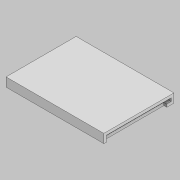
# Autodesk Inventor part: HardDriveCase
Saved by Autodesk Inventor 2021 (Build 250183000, 183)
## iProperties
Created: 2021-03-03
Part Number: HardDriveCase
Material: Generic
Document SubType Name: Modeling
Designer: Merkileg
Density: 1 g/cm^3
Appearance: Default
Author: Merkileg
Autodesk Inventor part; units mm, degrees
ref_plane "YZ Plane" through (0, 0, 0) normal (1, 0, 0) x (0, 1, 0)
ref_plane "XZ Plane" through (0, 0, 0) normal (0, 1, 0) x (-1, 0, 0)
ref_plane "XY Plane" through (0, 0, 0) normal (0, 0, 1) x (1, 0, 0)
sketch "Sketch1" plane through (0, 0, 0) normal (1, 0, 0) x (0, 1, 0)
  line L0 (0, 0) -> (9.779, 0)
  line L1 (9.779, 0) -> (9.779, -77.47)
  line L2 (9.779, -77.47) -> (0, -77.47)
  line L3 (0, -77.47) -> (0, 0)
  line L4 (3.175, -3.175) -> (6.604, -3.175)
  line L5 (6.604, -3.175) -> (6.604, -74.295)
  line L6 (6.604, -74.295) -> (3.175, -74.295)
  line L7 (3.175, -74.295) -> (3.175, -3.175)
  dimension "d0" = 3.175
  dimension "d1" = 3.175
  dimension "d2" = 3.175
  dimension "d3" = 3.175
  dimension "d4" = 3.429
  dimension "d5" = 71.12
  constraints: 16 end point, 4 parallel, 2 horizontal, 2 perpendicular
  measures "d0" distance between parallel lines of L1 L5
  measures "d1" distance between parallel lines of L2 L6
  measures "d2" distance between parallel lines of L0 L4
  measures "d3" distance between parallel lines of L7 L3
  measures "d4" distance between parallel lines of L7 L5
  measures "d5" distance between parallel lines of L6 L4
extrude "Extrusion1" add sketch "Sketch1" along normal blind 104.902
sketch "Sketch2" plane through (0, 0, 0) normal (-1, 0, 0) x (0, 0, 1)
  line L0 (-77.47, 0) -> (-77.47, 9.779) projected
  line L1 (0, 9.779) -> (0, 0) projected
  line L2 (-77.47, 9.779) -> (0, 9.779)
  line L3 (0, 9.779) -> (0, 0)
  line L4 (0, 0) -> (-77.47, 0)
  line L5 (-77.47, 0) -> (-77.47, 9.779)
  constraints: 8 end point, 2 parallel, 1 horizontal, 1 perpendicular
extrude "Extrusion2" add sketch "Sketch2" along normal blind 3.175
sketch "Sketch3" plane through (104.902, 0, 0) normal (1, 0, 0) x (0, 0, -1)
  line L0 (0, 0) -> (77.47, 0) projected
  line L1 (69.5325, 6.604) -> (2.8575, 6.604)
  line L2 (2.8575, 6.604) -> (2.8575, 0)
  line L3 (2.8575, 0) -> (69.5325, 0)
  line L4 (69.5325, 0) -> (69.5325, 6.604)
  line L5 (77.47, 0) -> (77.47, 9.779) projected
  dimension "d10" = 7.9375
  dimension "d11" = 66.675
  constraints: 8 end point, 2 parallel, 1 horizontal, 1 perpendicular, 1 point on line
  measures "d10" distance between parallel lines of L4 L5
  measures "d11" distance between parallel lines of L2 L4
extrude "Extrusion3" cut sketch "Sketch3" against normal blind 3.175
body "Solid1"
